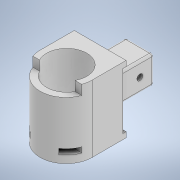
# Autodesk Inventor part: 5_Connettore_sup_inf
Saved by Autodesk Inventor 2020.2 (Build 242310000, 310)
## iProperties
Created: 2019-10-13
Part Number: 5_Connettore_sup_inf
Material: PLA(Stampato)
Document SubType Name: Modeling
Designer: socci
Density: 0.988 g/cm^3
Appearance: Default(1)
Mass: 64.0108 g
Surface Area: 242.78 cm^2
Volume: 64.7882 cm^3
Author: socci
Autodesk Inventor part; units mm, degrees
ref_plane "YZ Plane" through (0, 0, 0) normal (1, 0, 0) x (0, 1, 0)
ref_plane "XZ Plane" through (0, 0, 0) normal (0, 1, 0) x (-1, 0, 0)
ref_plane "XY Plane" through (0, 0, 0) normal (0, 0, 1) x (1, 0, 0)
sketch "Schizzo1" plane through (0, 0, 0) normal (0, 0, 1) x (1, 0, 0)
  line L0 (9, 6) -> (9, -6)
  line L1 (6, -9) -> (-6, -9)
  line L2 (-9, -6) -> (-9, 6)
  line L3 (-6, 9) -> (6, 9)
  arc A0 (-6, 9) -> (-9, 6) centre (-6, 6) ccw
  arc A1 (-9, -6) -> (-6, -9) centre (-6, -6) ccw
  arc A2 (6, -9) -> (9, -6) centre (6, -6) ccw
  arc A3 (9, 6) -> (6, 9) centre (6, 6) ccw
  point P0 (0, 0)
  point P1 (0, 0)
  point P2 (9, 9)
  point P3 (9, -9)
  point P4 (-9, -9)
  point P5 (-9, 9)
  dimension "d0" = 18
  dimension "d72" = 3
  constraints: 8 end point, 8 point on circle, 8 point on line, 8 tangent, 4 centre point, 3 equal radius, 1 coincident, 9 other
  measures "d0" distance of point (9, 9) point (9, -9)
  measures "d72" radius of A0
extrude "Estrusione1" add sketch "Schizzo1" against normal blind 40
sketch "Schizzo2" plane through (0, 0, 0) normal (0, 0, 1) x (1, 0, 0)
  line L0 (24.2, -31.25) -> (-24.2, -31.25)
  line L1 (-24.2, -31.25) -> (-24.2, 31.25)
  line L2 (-24.2, 31.25) -> (24.2, 31.25)
  line L3 (24.2, 31.25) -> (24.2, -31.25)
  line L4 (24.2, -31.25) -> (-24.2, 31.25) construction
  line L5 (-24.2, -31.25) -> (24.2, 31.25) construction
  point P0 (0, 0)
  dimension "d3" = 62.5
  dimension "d4" = 48.4
  constraints: 12 end point, 3 midpoint, 2 parallel, 1 horizontal, 1 perpendicular
  measures "d3" distance of L0.end L1.end
  measures "d4" distance of L1.end L2.end
extrude "Estrusione2" add sketch "Schizzo2" along normal blind 53
sketch "Schizzo3" plane through (-24.2, 31.25, 0) normal (0, 1, 0) x (1, 0, 0)
  line L0 (24.2, 0) -> (24.2, -28.2)
  line L1 (24.2, 0) -> (52.4, 0) construction
  circle A0 centre (24.2, -28.2) radius 18.75
  dimension "d7" = 28.2
  dimension "d8" = 90
  dimension "d9" = 37.5
  constraints: 4 end point, 1 centre point, 1 coincident, 1 horizontal, 1 perpendicular, 1 vertical
  measures "d7" distance of L0.start L0.end
  measures "d8" angle of L0 L1
  measures "d9" diameter of A0
extrude "Estrusione3" cut sketch "Schizzo3" against normal blind 55.5
sketch "Schizzo14" plane through (0, 0, 0) normal (0, 0, -1) x (-1, 0, 0)
  line L0 (-11, 13) -> (11, 13)
  line L1 (13, 11) -> (13, -11)
  line L2 (11, -13) -> (-11, -13)
  line L3 (-13, -11) -> (-13, 11)
  arc A0 (11, -13) -> (13, -11) centre (11, -11) ccw
  arc A1 (-13, -11) -> (-11, -13) centre (-11, -11) ccw
  arc A2 (13, 11) -> (11, 13) centre (11, 11) ccw
  arc A3 (-11, 13) -> (-13, 11) centre (-11, 11) ccw
  line L4 (-9.382, 10.5) -> (9.382, 10.5)
  line L5 (10.5, 9.382) -> (10.5, -9.382)
  line L6 (9.382, -10.5) -> (-9.382, -10.5)
  line L7 (-10.5, -9.382) -> (-10.5, 9.382)
  arc A4 (-10.1273, 10.8333) -> (-10.8333, 10.1273) centre (-10.5, 10.5) ccw
  arc A5 (-10.1273, 10.8333) -> (-9.382, 10.5) centre (-9.382, 11.5) ccw
  arc A6 (-10.5, 9.382) -> (-10.8333, 10.1273) centre (-11.5, 9.382) ccw
  arc A7 (10.8333, 10.1273) -> (10.1273, 10.8333) centre (10.5, 10.5) ccw
  arc A8 (9.382, 10.5) -> (10.1273, 10.8333) centre (9.382, 11.5) ccw
  arc A9 (10.8333, 10.1273) -> (10.5, 9.382) centre (11.5, 9.382) ccw
  arc A10 (10.1273, -10.8333) -> (10.8333, -10.1273) centre (10.5, -10.5) ccw
  arc A11 (10.1273, -10.8333) -> (9.382, -10.5) centre (9.382, -11.5) ccw
  arc A12 (10.5, -9.382) -> (10.8333, -10.1273) centre (11.5, -9.382) ccw
  arc A13 (-10.8333, -10.1273) -> (-10.1273, -10.8333) centre (-10.5, -10.5) ccw
  arc A14 (-9.382, -10.5) -> (-10.1273, -10.8333) centre (-9.382, -11.5) ccw
  arc A15 (-10.8333, -10.1273) -> (-10.5, -9.382) centre (-11.5, -9.382) ccw
  point P0 (0, 0)
  point P1 (0, 0)
  point P2 (-10.5, 10.5)
  point P3 (10.5, 10.5)
  point P4 (10.5, -10.5)
  point P5 (-10.5, -10.5)
  point P6 (0, 0)
  point P7 (-13, 13)
  point P8 (13, 13)
  point P9 (13, -13)
  point P10 (-13, -13)
  point P11 (0, 0)
  point P12 (-10, 10.5)
  point P13 (-10.5, 10)
  point P14 (10.5, 10)
  point P15 (10, 10.5)
  point P16 (10, -10.5)
  point P17 (10.5, -10)
  point P18 (-10.5, -10)
  point P19 (-10, -10.5)
  dimension "d77" = 21
  dimension "d78" = 26
  dimension "d102" = 2
  dimension "d110" = 1
  dimension "d112" = 1
  dimension "d114" = 1
  dimension "d116" = 1
  constraints: 40 point on circle, 24 tangent, 16 centre point, 16 end point, 16 point on line, 5 equal radius, 3 coincident, 19 other
  measures "d77" distance of point (-10.5, -10.5) point (-10.5, 10.5)
  measures "d78" distance of point (-13, -13) point (-13, 13)
  measures "d102" radius of A2
  measures "d110" radius of A5
  measures "d112" radius of A8
  measures "d114" radius of A11
  measures "d116" radius of A14
extrude "Estrusione10" add sketch "Schizzo14" along normal blind 40
sketch "Schizzo15" plane through (-13, 13, 0) normal (0, 1, 0) x (1, 0, 0)
  line L0 (13, 0) -> (13, 13)
  line L1 (13, 0) -> (26, 0) construction
  dimension "d82" = 13
  dimension "d83" = 90
  constraints: 4 end point, 1 horizontal, 1 perpendicular, 1 vertical
  measures "d82" distance of L0.start L0.end
  measures "d83" angle of L1 L0
hole "Foro4" at (0, 13, -13) direction (0, -1, 0) diameter 5.5 depth 26 tip angle 118 clearance for "Vite a testa esagonale" size "M5" standard "ANSI - Profilo M Metrico"
sketch "Schizzo16" plane through (13, -11, 0) normal (1, 0, 0) x (0, 0, -1)
  line L0 (0, 11) -> (27, 11)
  line L1 (0, 11) -> (27, 11) construction
  dimension "d91" = 27
  dimension "d92" = 0
  constraints: 4 end point, 2 horizontal, 1 collinear
  measures "d91" distance of L0.start L0.end
  measures "d92" distance between parallel lines of L0 L1
hole "Foro5" at (13, 0, -27) direction (-1, 0, 0) diameter 5.5 depth 26 tip angle 118 clearance for "Vite a testa esagonale" size "M5" standard "ANSI - Profilo M Metrico"
fillet "Raccordo1" radius 2 1 edges at (0, -13, -40)
fillet "Raccordo2" radius 2 1 edges at (-9, 0, -40)
fillet "Raccordo3" radius 6 1 edges at (-13, 0, 0)
sketch "Schizzo26" plane through (-24.2, -31.25, 0) normal (0, -1, 0) x (1, 0, 0)
  circle A0 centre (24.2, 28.2) radius 18.75 projected
  line L0 (24.2, 46.95) -> (24.2, 27.55)
  line L1 (24.2, 46.95) -> (43.6, 46.95) construction
  line L2 (24.2, 27.55) -> (24.2, 21.55)
  circle A1 centre (24.2, 21.55) radius 6.4
  point P0 (24.2, 0)
  dimension "d159" = 19.4
  dimension "d160" = 90
  dimension "d161" = 6
  dimension "d162" = 180
  dimension "d163" = 12.8
  constraints: 6 end point, 1 centre point, 1 coincident, 1 collinear, 1 horizontal, 1 perpendicular, 1 vertical, 1 vertical alignment, 1 other
  measures "d159" distance of L0.start L0.end
  measures "d160" angle of L0 L1
  measures "d161" distance of L0.end L2.end
  measures "d162" angle of L2 L0
  measures "d163" diameter of A1
extrude "Estrusione16" cut sketch "Schizzo26" against normal blind 10 contours A1
sketch "Schizzo27" plane through (-24.2, -31.25, 0) normal (0, -1, 0) x (1, 0, 0)
  circle A0 centre (24.2, 28.2) radius 18.75 projected
  line L0 (24.2, 28.2) -> (39.5, 28.2)
  point P0 (24.2, 0)
  point P1 (31.85, 41.4502)
  point P2 (16.55, 41.4502)
  point P3 (8.9, 28.2)
  point P4 (16.55, 14.9498)
  point P5 (31.85, 14.9498)
  dimension "d166" = 15.3
  dimension "d169" = 360
  constraints: 2 end point, 1 coincident, 1 horizontal, 7 other
  measures "d166" distance of L0.start L0.end
hole "Foro9" at (-15.3, -31.25, 28.2) at (-7.65, -31.25, 41.4502) at (7.65, -31.25, 41.4502) at (15.3, -31.25, 28.2) direction (0, 1, 0) diameter 3.8 depth 8.8 tip angle 118 clearance for "Vite a testa svasata piana ISO 2009/7046" size "M3" standard "ISO"
sketch "Schizzo28" plane through (-24.2, -31.25, 0) normal (-1, 0, 0) x (0, 0, 1)
  line L0 (53, 62.5) -> (53, 0) projected
  line L1 (53, 0) -> (53, 7)
  line L2 (53, 0) -> (60, 0) construction
  line L3 (53, 7) -> (53, 12)
  line L4 (53, 7) -> (53, 12)
  line L5 (53, 12) -> (37, 12)
  line L6 (53, 12) -> (49.5, 12)
  line L7 (53, 12) -> (56.5, 12) construction
  line L8 (53, 12) -> (49, 12)
  line L9 (37, 12) -> (37, 7)
  line L10 (37, 12) -> (42, 12) construction
  line L11 (37, 7) -> (49, 7)
  line L12 (49, 7) -> (49, 12)
  line L13 (49, 12) -> (37, 12)
  line L14 (37, 12) -> (37, 7)
  line L15 (53, 62.5) -> (53, 53.5)
  line L16 (53, 62.5) -> (62, 62.5) construction
  line L17 (53, 62.5) -> (53, 53.5)
  line L18 (53, 53.5) -> (37, 53.5)
  line L19 (37, 53.5) -> (37, 62.5)
  line L20 (37, 62.5) -> (53, 62.5)
  point P0 (0, 31.25)
  dimension "d178" = 7
  dimension "d179" = 90
  dimension "d180" = 5
  dimension "d181" = 180
  dimension "d184" = 180
  dimension "d185" = 4
  dimension "d186" = 5
  dimension "d187" = 90
  dimension "d188" = 9
  dimension "d189" = 90
  dimension "d190" = 16
  constraints: 40 end point, 6 horizontal, 4 collinear, 4 equal length, 4 parallel, 3 perpendicular, 2 vertical, 1 point on line
  measures "d178" distance of L0.end L1.end
  measures "d179" angle of L2 L1
  measures "d180" distance of L1.end L3.end
  measures "d181" angle of L3 L1
  measures "d184" angle of L6 L7
  measures "d185" distance of L3.end L8.end
  measures "d186" distance of L5.end L9.end
  measures "d187" angle of L9 L10
  measures "d188" distance of L0.start L15.end
  measures "d189" angle of L15 L16
  measures "d190" distance of L15.end L18.end
extrude "Estrusione17" cut sketch "Schizzo28" against normal through all
full round fillet "Raccordo5" first side at (24.2, -6.4167, 12.3333) centre faces at (8.0667, -13.4167, 53) second side at (-24.2, -6.4167, 12.3333)
sketch "Schizzo29" plane through (0, 0, 0) normal (0, 0, -1) x (-1, 0, 0)
  line L0 (-24.2, -31.25) -> (-24.2, 31.25) projected
  line L1 (-24.2, -31.25) -> (-24.2, -26.25)
  line L2 (-24.2, -31.25) -> (-19.2, -31.25) construction
  line L3 (24.2, -31.25) -> (-24.2, -31.25) projected
  line L4 (24.2, -31.25) -> (-24.2, -31.25)
  line L5 (-24.2, -31.25) -> (-24.2, -26.25)
  line L6 (-24.2, -26.25) -> (24.2, -26.25)
  line L7 (24.2, -26.25) -> (24.2, -31.25)
  line L8 (-24.2, 31.25) -> (-24.2, 26.25)
  line L9 (-24.2, 31.25) -> (-19.2, 31.25) construction
  line L10 (24.2, 31.25) -> (-24.2, 31.25)
  line L11 (-24.2, 31.25) -> (-24.2, 26.25)
  line L12 (-24.2, 26.25) -> (24.2, 26.25)
  line L13 (24.2, 26.25) -> (24.2, 31.25)
  point P0 (0, 0)
  dimension "d193" = 5
  dimension "d194" = 90
  dimension "d195" = 5
  dimension "d196" = 90
  constraints: 24 end point, 5 perpendicular, 4 parallel, 3 collinear, 2 horizontal
  measures "d193" distance of L0.start L1.end
  measures "d194" angle of L2 L1
  measures "d195" distance of L0.end L8.end
  measures "d196" angle of L8 L9
extrude "Estrusione18" add sketch "Schizzo29" along normal blind 3
